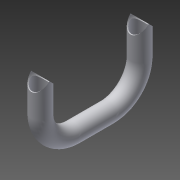
# Autodesk Inventor part: Rura_pozioma_podnóżka
Saved by Autodesk Inventor 2015 (Build 190159000, 159)
## iProperties
Created: 2015-12-07
Part Number: Rura_pozioma_podnóżka
Material: Aluminium AW-7020
Document SubType Name: Modeling
Designer: graaapsik
Density: 2.78 g/cm^3
Appearance: Aluminium AW-7020
Author: graaapsik
Autodesk Inventor part; units mm, degrees
ref_plane "YZ Plane" through (0, 0, 0) normal (1, 0, 0) x (0, 1, 0)
ref_plane "XZ Plane" through (0, 0, 0) normal (0, 1, 0) x (-1, 0, 0)
ref_plane "XY Plane" through (0, 0, 0) normal (0, 0, 1) x (1, 0, 0)
ref_plane "Płaszczyzna konstrukcyjna1" through (520, 0, 14) normal (0, 0, -1) x (-1, 0.0000001, 0)
sketch "Szkic1" plane through (520, 0, 14) normal (0, 0, -1) x (-1, 0.0000001, 0)
  circle A0 centre (260, 244.3579) radius 14
  circle A1 centre (260, 244.3579) radius 12.5
  line L0 (274, 168.3579) -> (223.2217, 168.3579) construction
  circle A2 centre (260, 92.3579) radius 14 construction
  line L1 (274, 261.7157) -> (274, 75) construction
  point P0 (520, 0)
  dimension "d0" = 28
  dimension "d1" = 1.5
  dimension "d3" = 152
  constraints: 4 end point, 3 centre point, 1 midpoint, 1 tangent, 1 vertical, 1 vertical alignment, 3 other
  measures "d0" diameter of A0
  measures "d1" radial gap between concentric circles of A1 A0
  measures "d3" distance of A2.centre A0.centre
ref_plane "Płaszczyzna konstrukcyjna2" through (246, 0, 14) normal (1, 0, 0) x (0, 1, 0)
sketch "Szkic2" plane through (246, 0, 14) normal (1, 0, 0) x (0, 1, 0)
  line L0 (78.3579, 0) -> (106.3579, 0) construction
  line L1 (230.3579, 0) -> (258.3579, 0) projected
  line L2 (92.3579, 0) -> (92.3579, -49)
  line L3 (142.3579, -99) -> (194.3579, -99)
  line L4 (244.3579, -49) -> (244.3579, 0)
  arc A0 (92.3579, -49) -> (142.3579, -99) centre (142.3579, -49) ccw
  arc A1 (194.3579, -99) -> (244.3579, -49) centre (194.3579, -49) ccw
  point P0 (0, -14)
  point P1 (92.3579, -99)
  dimension "d4" = 99
  dimension "d5" = 50
  constraints: 6 end point, 4 point on circle, 4 tangent, 2 centre point, 2 midpoint, 2 perpendicular, 2 point on line, 1 equal radius, 1 vertical
  measures "d4" distance of L2.start point (92.358, -99)
  measures "d5" radius of A0
sweep "Przeciągnięcie1" add profiles "Szkic1" path "Szkic2" path curves L4 A1 L3 A0 L2
sketch "Szkic3" plane through (0, 0, 0) normal (0, 1, 0) x (-1, 0, 0)
  line L0 (-246, 14) -> (-274, 14) construction
  circle A0 centre (-260, 14) radius 14
  point P0 (0, 0)
  dimension "d7" = 28
  constraints: 1 centre point, 1 midpoint
  measures "d7" diameter of A0
extrude "Wyciągnięcie proste1" add sketch "Szkic3" along normal blind 274.5 separate body
combine bodies "Utwórz kombinację1" operation type subtract main body 1 bodies to subtract 2
